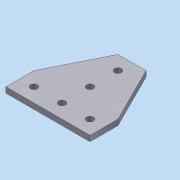
# Autodesk Inventor part: 5 Hole T Joining Plate
Saved by Autodesk Inventor 2015 (Build 190159000, 159)
## iProperties
Created: 2013-12-08
Part Number: 5 Hole T Joining Plate
Material: Aluminum 6061
Document SubType Name: Modeling
Designer: OpenBuilds
Density: 2.71 g/cm^3
Catalog Web Link: www.openbuildspartstore.com
Vendor: OpenBuilds
Mass: 29.2878 g
Surface Area: 65.5558 cm^2
Volume: 10.8073 cm^3
Appearance: Aluminum - Flat
Author: Work
Autodesk Inventor part; units mm, degrees
ref_plane "YZ Plane" through (0, 0, 0) normal (1, 0, 0) x (0, 1, 0)
ref_plane "XZ Plane" through (0, 0, 0) normal (0, 1, 0) x (-1, 0, 0)
ref_plane "XY Plane" through (0, 0, 0) normal (0, 0, 1) x (1, 0, 0)
sketch "Sketch1" plane through (0, 0, 0) normal (0, 0, 1) x (1, 0, 0)
  line L0 (30, 10) -> (-30, 10) construction
  line L1 (-30, 10) -> (-30, -10) construction
  line L2 (-30, -10) -> (30, -10) construction
  line L3 (30, -10) -> (30, 10) construction
  line L4 (30, 10) -> (-30, -10) construction
  line L5 (-30, 10) -> (30, -10) construction
  line L6 (-10, 50) -> (10, 50) construction
  line L7 (10, 50) -> (10, -10) construction
  line L8 (10, -10) -> (-10, -10) construction
  line L9 (-10, -10) -> (-10, 50) construction
  line L10 (-10, 50) -> (10, -10) construction
  line L11 (10, 50) -> (-10, -10) construction
  line L12 (-10, 50) -> (10, 50)
  line L13 (10, 50) -> (30, 10)
  line L14 (30, 10) -> (30, -10)
  line L15 (30, -10) -> (-30, -10)
  line L16 (-30, -10) -> (-30, 10)
  line L17 (-30, 10) -> (-10, 50)
  line L18 (0, 20) -> (0, 0) construction
  dimension "d0" = 20
  dimension "d2" = 20
  dimension "d3" = 60
  dimension "d4" = 60
  constraints: 38 end point, 8 equal length, 4 midpoint, 3 perpendicular, 2 horizontal, 1 point on line
  measures "d0" distance of L6.start L6.end
  measures "d2" distance of L0.end L1.end
  measures "d3" distance of L1.end L2.end
  measures "d4" distance between parallel lines of L2 L6
extrude "Extrusion1" add sketch "Sketch1" along normal mid plane 4
sketch "Sketch2" plane through (0, 0, 2) normal (0, 0, 1) x (1, 0, 0)
  line L0 (10, 50) -> (-10, 50) construction
  line L1 (-30, 10) -> (-30, -10) construction
  line L2 (-30, -10) -> (30, -10) construction
  line L3 (30, -10) -> (30, 10) construction
  line L4 (30, 0) -> (-30, 0) construction
  line L5 (0, 50) -> (0, -10) construction
  point P0 (0, 0)
  point P1 (0, 0)
  point P2 (-20, 0)
  point P3 (20, 0)
  point P4 (0, 20)
  point P5 (0, 40)
  dimension "d7" = 40
  dimension "d9" = 20
  dimension "d10" = 20
  dimension "d11" = 20
  constraints: 5 midpoint, 4 end point, 3 point on line, 1 coincident
  measures "d7" distance of point (20, 0) point (-20, 0)
  measures "d9" distance of point (0, 0) point (-20, 0)
  measures "d10" distance of point (0, 0) point (0, 20)
  measures "d11" distance of point (0, 20) point (0, 40)
hole "Hole1" at (0, 0, 2) at (-20, 0, 2) at (20, 0, 2) at (0, 20, 2) at (0, 40, 2) direction (0, 0, -1) diameter 5 end through all
body "Solid1"
